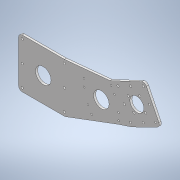
# Autodesk Inventor part: 関節3_側板左
Saved by Autodesk Inventor 2021 (Build 250183000, 183)
## iProperties
Created: 2022-02-03
Part Number: 関節3_側板左
Material: 一般
Document SubType Name: Modeling
Designer: hirohumi
Density: 1 g/cm^3
Appearance: 既定
Author: hirohumi
Autodesk Inventor part; units mm, degrees
ref_plane "YZ Plane" through (0, 0, 0) normal (1, 0, 0) x (0, 1, 0)
ref_plane "XZ Plane" through (0, 0, 0) normal (0, 1, 0) x (-1, 0, 0)
ref_plane "XY Plane" through (0, 0, 0) normal (0, 0, 1) x (1, 0, 0)
sketch "スケッチ1" plane through (0, 0, 0) normal (0, 0, 1) x (1, 0, 0)
  circle A0 centre (0, 0) radius 11.05
  line L0 (30, 30) -> (-30, 30) construction
  line L1 (-30, 30) -> (-30, -30) construction
  line L2 (-30, -30) -> (30, -30) construction
  line L3 (30, -30) -> (30, 30) construction
  line L4 (30, 30) -> (-30, -30) construction
  line L5 (-30, 30) -> (30, -30) construction
  circle A1 centre (-30, 30) radius 1.6
  circle A2 centre (30, 30) radius 1.6
  circle A3 centre (30, -30) radius 1.6
  circle A4 centre (-30, -30) radius 1.6
  circle A5 centre (-30, 0) radius 1.6
  circle A6 centre (30, 0) radius 1.6
  circle A7 centre (0, 300) radius 10 construction
  line L6 (0, 300) -> (82.4797, 11.5609) construction
  line L7 (0, 300) -> (132.9888, 31.0874) construction
  arc A8 (0, 0) -> (244.9763, 126.8336) centre (0, 300) ccw construction
  line L8 (106.8619, 8.1323) -> (101.3633, 27.3615) construction
  circle A9 centre (82.4797, 11.5609) radius 11.05
  line L9 (96.2103, 36.2888) -> (57.7518, 25.2915) construction
  line L10 (101.3633, 27.3615) -> (58.0974, 14.9896) construction
  line L11 (58.0974, 14.9896) -> (106.8619, 8.1323) construction
  line L12 (101.3633, 27.3615) -> (63.5961, -4.2397) construction
  line L13 (63.5961, -4.2397) -> (106.8619, 8.1323) construction
  line L14 (96.2103, 36.2888) -> (68.7491, -13.167) construction
  circle A10 centre (82.4797, 11.5609) radius 23.5 construction
  line L15 (68.7491, -13.167) -> (107.2076, -2.1697) construction
  circle A11 centre (63.5961, -4.2397) radius 1.25
  line L16 (58.0974, 14.9896) -> (63.5961, -4.2397) construction
  line L17 (57.7518, 25.2915) -> (68.7491, -13.167) construction
  circle A12 centre (101.3633, 27.3615) radius 1.25
  circle A13 centre (101.3633, 27.3615) radius 5 construction
  circle A14 centre (107.2076, -2.1697) radius 1.25
  arc A15 (111.2054, -2.0356) -> (105.4181, -5.7471) centre (107.2076, -2.1697) ccw construction
  circle A16 centre (68.7491, -13.167) radius 1.25
  circle A17 centre (57.7518, 25.2915) radius 1.25
  circle A18 centre (106.8619, 8.1323) radius 1.25
  line L18 (107.2076, -2.1697) -> (96.2103, 36.2888) construction
  circle A19 centre (58.0974, 14.9896) radius 1.25
  circle A20 centre (96.2103, 36.2888) radius 1.25
  circle A21 centre (58.0974, 14.9896) radius 5 construction
  line L19 (57.7518, 25.2915) -> (107.2076, -2.1697) construction
  line L20 (37.5, 43.7095) -> (22.5, 43.7095) construction
  line L21 (22.5, 43.7095) -> (22.5, -43.7095) construction
  line L22 (22.5, -43.7095) -> (37.5, -43.7095) construction
  line L23 (37.5, -43.7095) -> (37.5, 43.7095) construction
  line L24 (37.5, 43.7095) -> (22.5, -43.7095) construction
  line L25 (22.5, 43.7095) -> (37.5, -43.7095) construction
  circle A22 centre (132.9888, 31.0874) radius 23 construction
  arc A23 (-30, 35) -> (-35, 30) centre (-30, 30) ccw
  arc A24 (-35, -30) -> (-30, -35) centre (-30, -30) ccw
  arc A25 (30, -35) -> (31.7527, -34.6827) centre (30, -30) ccw
  arc A26 (100.5407, 38.7884) -> (95.7358, 41.2663) centre (96.2103, 36.2888) ccw construction
  line L26 (108.5253, -5.9475) -> (31.7527, -34.6827)
  line L27 (30, -35) -> (-30, -35)
  line L28 (-35, -30) -> (-35, 30)
  line L29 (-30, 35) -> (30, 35)
  line L30 (30, 35) -> (94.8682, 41.1836)
  circle A27 centre (0, 0) radius 55 construction
  line L31 (142.0504, 57.8808) -> (106.1954, 40.149) construction
  line L32 (106.1954, 40.149) -> (123.9272, 4.294) construction
  line L33 (123.9272, 4.294) -> (159.7822, 22.0258) construction
  line L34 (159.7822, 22.0258) -> (142.0504, 57.8808) construction
  line L35 (142.0504, 57.8808) -> (123.9272, 4.294) construction
  line L36 (106.1954, 40.149) -> (159.7822, 22.0258) construction
  circle A28 centre (106.1954, 40.149) radius 1.6
  circle A29 centre (142.0504, 57.8808) radius 1.6
  circle A30 centre (159.7822, 22.0258) radius 1.6
  circle A31 centre (123.9272, 4.294) radius 1.6
  circle A32 centre (132.9888, 31.0874) radius 10
  circle A33 centre (120.674, 35.2523) radius 1.6
  circle A34 centre (137.1537, 43.4022) radius 1.6
  circle A35 centre (145.3036, 26.9225) radius 1.6
  circle A36 centre (128.8239, 18.7726) radius 1.6
  circle A37 centre (132.9888, 31.0874) radius 13 construction
  circle A38 centre (124.1229, 49.0149) radius 1.6
  circle A39 centre (141.8547, 13.1599) radius 1.6
  circle A40 centre (106.1954, 40.149) radius 5 construction
  arc A41 (126.1437, -0.1879) -> (125.4672, -0.463) centre (123.9272, 4.294) ccw construction
  line L37 (101.7135, 37.9325) -> (119.4454, 2.0775) construction
  arc A42 (146.5323, 60.0973) -> (139.9198, 62.4042) centre (142.0504, 57.8808) ccw
  arc A43 (161.9987, 17.544) -> (164.2641, 24.2423) centre (159.7822, 22.0258) ccw
  line L38 (139.9198, 62.4042) -> (94.8682, 41.1836)
  line L39 (146.5323, 60.0973) -> (164.2641, 24.2423)
  line L40 (161.9987, 17.544) -> (126.1437, -0.1879)
  line L41 (108.5253, -5.9475) -> (125.4672, -0.463)
  arc A44 (125.4672, -0.463) -> (126.1437, -0.1879) centre (123.9272, 4.294) ccw
  circle A45 centre (115.0613, 22.2215) radius 1.6
  circle A46 centre (150.9163, 39.9533) radius 1.6
  point P0 (82.4797, 11.5609)
  dimension "d59" = 10
  dimension "d0" = 22.1
  dimension "d1" = 60
  dimension "d2" = 60
  dimension "d3" = 3.2
  dimension "d5" = 3.2
  dimension "d6" = 3.2
  dimension "d8" = 3.2
  dimension "d9" = 3.2
  dimension "d10" = 3.2
  dimension "d11" = 20
  dimension "d13" = 300
  dimension "d14" = 47
  dimension "d15" = 22.1
  dimension "d16" = 20
  dimension "d17" = 45
  dimension "d18" = 40
  dimension "d19" = 40
  dimension "d20" = 2.5
  dimension "d21" = 2.5
  dimension "d22" = 2.5
  dimension "d23" = 2.5
  dimension "d24" = 2.5
  dimension "d25" = 2.5
  dimension "d26" = 2.5
  dimension "d27" = 2.5
  dimension "d28" = 10
  dimension "d30" = 8
  dimension "d31" = 10
  dimension "d32" = 15
  dimension "d33" = 46
  dimension "d35" = 5
  dimension "d38" = 5
  dimension "d39" = 5
  dimension "d40" = 5
  dimension "d41" = 5
  dimension "d44" = 110
  dimension "d45" = 40
  dimension "d46" = 40
  dimension "d47" = 3.2
  dimension "d48" = 3.2
  dimension "d49" = 3.2
  dimension "d50" = 3.2
  dimension "d51" = 20
  dimension "d52" = 3.2
  dimension "d53" = 3.2
  dimension "d54" = 3.2
  dimension "d55" = 3.2
  dimension "d56" = 13
  dimension "d57" = 3.2
  dimension "d58" = 3.2
  dimension "d60" = 10
  dimension "d61" = 5
  dimension "d62" = 5
  dimension "d65" = 3.2
  dimension "d66" = 3.2
  constraints: 85 end point, 46 centre point, 34 coincident, 27 point on circle, 20 midpoint, 17 tangent, 12 parallel, 8 perpendicular, 6 point on line, 2 horizontal, 1 vertical alignment, 4 other
  measures "d0" diameter of A0
  measures "d1" distance of L2.end L1.end
  measures "d2" distance of L1.end L0.end
  measures "d3" diameter of A1
  measures "d5" diameter of A2
  measures "d6" diameter of A3
  measures "d8" diameter of A4
  measures "d9" diameter of A5
  measures "d10" diameter of A6
  measures "d11" diameter of A7
  measures "d13" radius of A8
  measures "d14" diameter of A10
  measures "d15" diameter of A9
  measures "d16" distance of L11.start L13.start
  measures "d17" distance of L13.start L13.end
  measures "d18" distance of L15.start L15.end
  measures "d19" distance of L9.end L15.start
  measures "d20" diameter of A17
  measures "d21" diameter of A19
  measures "d22" diameter of A11
  measures "d23" diameter of A16
  measures "d24" diameter of A20
  measures "d25" diameter of A12
  measures "d26" diameter of A18
  measures "d27" diameter of A14
  measures "d28" diameter of A13
  measures "d30" diameter of A15
  measures "d31" diameter of A21
  measures "d32" distance of L22.end L21.end
  measures "d33" diameter of A22
  measures "d35" radius of A26
  measures "d38" radius of A23
  measures "d39" radius of A24
  measures "d40" radius of A25
  measures "d41" distance of L0.start L29.end
  measures "d44" diameter of A27
  measures "d45" distance of L33.end L32.end
  measures "d46" distance of L32.end L31.end
  measures "d47" diameter of A28
  measures "d48" diameter of A29
  measures "d49" diameter of A30
  measures "d50" diameter of A31
  measures "d51" diameter of A32
  measures "d52" diameter of A33
  measures "d53" diameter of A34
  measures "d54" diameter of A35
  measures "d55" diameter of A36
  measures "d56" distance of L7.end A34.centre
  measures "d57" diameter of A38
  measures "d58" diameter of A39
  measures "d60" diameter of A41
  measures "d61" radius of A42
  measures "d62" radius of A43
  measures "d65" diameter of A45
  measures "d66" diameter of A46
extrude "押し出し2" add sketch "スケッチ1" along normal blind 3
